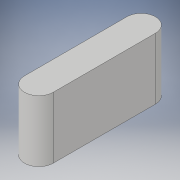
# Autodesk Inventor part: slot_6mm
Saved by Autodesk Inventor 2019 (Build 230136000, 136)
## iProperties
Created: 2019-05-07
Part Number: slot_6mm
Material: Generic
Document SubType Name: Modeling
Designer: assman
Density: 1 g/cm^3
Appearance: Default
Author: assman
## iProperties of the stored document slot_6mm_3DPrint.ipt
Created: 2019-05-07
Part Number: slot_6mm_3DPrint
Material: Generic
Document SubType Name: Modeling
Designer: assman
Density: 1 g/cm^3
Appearance: Default
Author: assman
Autodesk Inventor part; units mm, degrees
ref_plane "YZ Plane" through (0, 0, 0) normal (1, 0, 0) x (0, 1, 0)
ref_plane "XZ Plane" through (0, 0, 0) normal (0, 1, 0) x (-1, 0, 0)
ref_plane "XY Plane" through (0, 0, 0) normal (0, 0, 1) x (1, 0, 0)
sketch "Sketch1" plane through (0, 0, 0) normal (0, 1, 0) x (-1, 0, 0)
  line L0 (0, 5) -> (0, -5) construction
  line L1 (-1.475, 5) -> (-1.475, -5) construction
  line L2 (1.475, -5) -> (1.475, 5) construction
  arc A0 (1.475, 5) -> (-1.475, 5) centre (0, 5) ccw construction
  arc A1 (-1.475, -5) -> (1.475, -5) centre (0, -5) ccw construction
  line L3 (1.395, 5) -> (1.395, -5)
  arc A2 (-1.395, -5) -> (1.395, -5) centre (0, -5) ccw
  line L4 (-1.395, -5) -> (-1.395, 5)
  arc A3 (1.395, 5) -> (-1.395, 5) centre (0, 5) ccw
  point P0 (0, 0)
  dimension "d0" = 5
  dimension "d1" = 2.95
  dimension "d4" = 0.08
  constraints: 12 end point, 8 point on circle, 4 centre point, 4 tangent, 2 parallel, 1 midpoint, 1 vertical, 3 other
  measures "d0" distance of point (0, 0) L0.end
  measures "d1" diameter of A1
  measures "d4" distance between parallel lines of L2 L3
extrude "Extrusion1" add sketch "Sketch1" along normal blind 6
body "Solid1"
